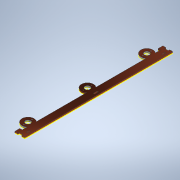
# Autodesk Inventor part: chassis_1_1
Saved by Autodesk Inventor 2022 (Build 260153000, 153)
## iProperties
Created: 2023-03-24
Part Number: chassis_1_1
Material: 一般
Document SubType Name: Modeling
Designer: Johnny Jou
Density: 1 g/cm^3
Appearance: 預設
Author: Johnny Jou
Autodesk Inventor part; units mm, degrees
ref_plane "YZ Plane" through (0, 0, 0) normal (1, 0, 0) x (0, 1, 0)
ref_plane "XZ Plane" through (0, 0, 0) normal (0, 1, 0) x (-1, 0, 0)
ref_plane "XY Plane" through (0, 0, 0) normal (0, 0, 1) x (1, 0, 0)
sketch "草圖1" plane through (0, 0, 0) normal (0, 1, 0) x (-1, 0, 0)
  line L0 (0, 0) -> (0, -306)
  arc A0 (15, -162.6047) -> (15, -143.3953) centre (23, -153) ccw
  circle A1 centre (23, -153) radius 26 construction
  line L1 (15, -296) -> (15, -162.6047)
  line L2 (15, -143.3953) -> (15, -10)
  circle A2 centre (23, -144.5) radius 1
  circle A3 centre (23, -161.5) radius 1
  line L3 (20, 0) -> (20, -10)
  line L4 (20, -10) -> (15, -10)
  line L5 (0, -10) -> (0, 0)
  line L6 (6, 0) -> (6, -3)
  line L7 (6, -3) -> (14, -3)
  line L8 (14, -3) -> (14, 0)
  line L9 (0, 0) -> (6, 0)
  line L10 (14, 0) -> (20, 0)
  line L11 (15, 0) -> (14, 0)
  line L12 (6, 0) -> (0, 0)
  line L13 (20, -306) -> (20, -296)
  line L14 (20, -296) -> (15, -296)
  line L15 (0, -290) -> (0, -306)
  line L16 (6, -306) -> (6, -303)
  line L17 (6, -303) -> (14, -303)
  line L18 (14, -303) -> (14, -306)
  line L19 (0, -306) -> (6, -306)
  line L20 (14, -306) -> (20, -306)
  dimension "d1" = 15
  dimension "d2" = 25
  dimension "d3" = 52
  dimension "d4" = 23
  dimension "d6" = 2
  dimension "d7" = 17
  dimension "d8" = 8.5
  dimension "d9" = 10
  dimension "d10" = 20
  dimension "d11" = 8
  dimension "d12" = 3
  dimension "d13" = 6
  dimension "d15" = 3
  dimension "d16" = 8
  dimension "d17" = 6
  dimension "d34" = 306
  dimension "d35" = 153
  dimension "d36" = 10
  dimension "d55" = 8.5
  constraints: 42 end point, 10 parallel, 6 horizontal, 6 perpendicular, 4 centre point, 2 coincident, 2 collinear, 2 point on circle, 1 equal radius, 1 vertical alignment
  measures "d1" distance of L11.start L0.start
  measures "d2" diameter of A0
  measures "d3" diameter of A1
  measures "d4" distance from line of L0 A0.centre
  measures "d6" diameter of A2
  measures "d7" distance of A3.centre A2.centre
  measures "d8" distance of A0.centre A3.centre
  measures "d9" distance of L3.start L3.end
  measures "d10" distance between parallel lines of L0 L3
  measures "d11" distance of L6.end L7.end
  measures "d12" distance of L7.end L8.end
  measures "d13" distance between parallel lines of L5 L6
  measures "d15" distance of L17.end L18.end
  measures "d16" distance of L16.end L17.end
  measures "d17" distance between parallel lines of L0 L16
  measures "d34" distance of L0.start L0.end
  measures "d35" distance from line of L19 A0.centre
  measures "d36" distance of L13.start L13.end
  measures "d55" distance of A0.centre A2.centre
extrude "擠出1" add sketch "草圖1" along normal blind 3
sketch "草圖2" plane through (0, 3, 0) normal (0, 1, 0) x (1, 0, 0)
  line L0 (-7, 149) -> (-4, 149)
  line L1 (-4, 149) -> (-4, 157)
  line L2 (-4, 157) -> (-7, 157)
  line L3 (-7, 157) -> (-7, 149)
  arc A0 (-15, 162.6047) -> (-15, 143.3953) centre (-23, 153) ccw projected
  line L4 (-15, 143.3953) -> (-15, 10) projected
  circle A1 centre (-23, 153) radius 12.5 construction
  line L5 (0, 0) -> (0, 306) projected
  line L6 (-7, 10) -> (-4, 10)
  line L7 (-4, 10) -> (-4, 16)
  line L8 (-4, 16) -> (-7, 16)
  line L9 (-7, 16) -> (-7, 10)
  line L10 (-14, 3) -> (-6, 3) projected
  line L11 (-7, 290) -> (-4, 290)
  line L12 (-4, 290) -> (-4, 296)
  line L13 (-4, 296) -> (-7, 296)
  line L14 (-7, 296) -> (-7, 290)
  line L15 (-6, 303) -> (-14, 303) projected
  dimension "d20" = 8
  dimension "d21" = 3
  dimension "d22" = 4
  dimension "d23" = 4
  dimension "d24" = 6
  dimension "d25" = 3
  dimension "d26" = 4
  dimension "d27" = 7
  dimension "d28" = 6
  dimension "d29" = 3
  dimension "d30" = 4
  dimension "d31" = 7
  constraints: 24 end point, 6 parallel, 3 horizontal, 3 perpendicular, 1 coincident, 3 other
  measures "d20" distance of L2.end L0.start
  measures "d21" distance of L1.end L2.end
  measures "d22" distance from line of A0.centre L2
  measures "d23" distance between parallel lines of L5 L1
  measures "d24" distance of L8.end L6.start
  measures "d25" distance of L7.end L8.end
  measures "d26" distance between parallel lines of L5 L7
  measures "d27" distance between parallel lines of L10 L6
  measures "d28" distance of L13.end L11.start
  measures "d29" distance of L11.start L11.end
  measures "d30" distance between parallel lines of L5 L12
  measures "d31" distance between parallel lines of L15 L13
extrude "擠出2" cut sketch "草圖2" against normal up to surface (3 mm away)
sketch "草圖3" plane through (0, 3, 0) normal (0, 1, 0) x (1, 0, 0)
  arc A0 (-15, 162.6047) -> (-15, 143.3953) centre (-23, 153) ccw projected
  circle A1 centre (-23, 153) radius 5.5
  point P0 (0, 0)
  dimension "d37" = 11
  constraints: 1 centre point, 1 coincident
  measures "d37" diameter of A1
extrude "擠出3" cut sketch "草圖3" against normal up to surface (3 mm away)
sketch "草圖4" plane through (0, 3, 0) normal (0, 1, 0) x (1, 0, 0)
  circle A0 centre (-23, 153) radius 5.5 projected
  arc A1 (-15, 162.6047) -> (-15, 143.3953) centre (-23, 153) ccw projected
  circle A2 centre (-23, 144.5) radius 1 projected
  circle A3 centre (-23, 161.5) radius 1 projected
  circle A4 centre (-23, 30) radius 12.5
  circle A5 centre (-23, 30) radius 5.5
  circle A6 centre (-23, 38.5) radius 1
  circle A7 centre (-23, 21.5) radius 1
  line L0 (-15, 143.3953) -> (-15, 10) projected
  circle A8 centre (-23, 276) radius 12.5
  circle A9 centre (-23, 276) radius 5.5
  circle A10 centre (-23, 284.5) radius 1
  circle A11 centre (-23, 267.5) radius 1
  point P0 (0, 0)
  point P1 (-15, 20.3953)
  point P2 (-15, 39.6047)
  dimension "d40" = 2
  dimension "d41" = 11
  dimension "d42" = 25
  dimension "d43" = 17
  dimension "d44" = 8.5
  dimension "d45" = 123
  dimension "d48" = 246
  constraints: 8 centre point, 3 vertical alignment, 2 coincident, 1 equal radius, 1 vertical, 8 other
  measures "d40" diameter of A6
  measures "d41" diameter of A5
  measures "d42" diameter of A4
  measures "d43" distance of A7.centre A6.centre
  measures "d44" distance of A4.centre A6.centre
  measures "d45" distance of A0.centre A4.centre
  measures "d48" distance of A4.centre A8.centre
extrude "擠出4" add sketch "草圖4" against normal up to surface (3 mm away) contours L0 A4 | A8 picked at (-15.8333, 30)
sketch "草圖5" plane through (0, 0, 0) normal (0, -1, 0) x (1, 0, 0)
  circle A0 centre (-23, -267.5) radius 1 projected
  circle A1 centre (-23, -284.5) radius 1 projected
  circle A2 centre (-23, -276) radius 5.5 projected
  circle A3 centre (-23, -21.5) radius 1 projected
  circle A4 centre (-23, -38.5) radius 1 projected
  circle A5 centre (-23, -30) radius 5.5 projected
  circle A6 centre (-23, -161.5) radius 1 projected
  circle A7 centre (-23, -144.5) radius 1 projected
  line L0 (-15, -296) -> (-15, -285.6047) projected
  line L1 (-20, -296) -> (-15, -296) projected
  line L2 (-20, -306) -> (-20, -296) projected
  line L3 (-14, -306) -> (-20, -306) projected
  line L4 (-14, -303) -> (-14, -306) projected
  line L5 (-6, -303) -> (-14, -303) projected
  line L6 (-6, -306) -> (-6, -303) projected
  line L7 (0, -306) -> (-6, -306) projected
  line L8 (0, 0) -> (0, -306) projected
  line L9 (-6, 0) -> (0, 0) projected
  line L10 (-6, -3) -> (-6, 0) projected
  line L11 (-14, -3) -> (-6, -3) projected
  line L12 (-14, 0) -> (-14, -3) projected
  line L13 (-20, 0) -> (-14, 0) projected
  line L14 (-20, -10) -> (-20, 0) projected
  line L15 (-15, -10) -> (-20, -10) projected
  line L16 (-15, -20.3953) -> (-15, -10) projected
  arc A8 (-15, -20.3953) -> (-15, -39.6047) centre (-23, -30) ccw projected
  line L17 (-15, -143.3953) -> (-15, -39.6047) projected
  arc A9 (-15, -143.3953) -> (-15, -162.6047) centre (-23, -153) ccw projected
  line L18 (-15, -266.3953) -> (-15, -162.6047) projected
  arc A10 (-15, -266.3953) -> (-15, -285.6047) centre (-23, -276) ccw projected
  line L19 (-7, -149) -> (-4, -149) projected
  line L20 (-4, -149) -> (-4, -157) projected
  line L21 (-4, -157) -> (-7, -157) projected
  line L22 (-7, -157) -> (-7, -149) projected
  line L23 (-4, -10) -> (-4, -16) projected
  line L24 (-4, -16) -> (-7, -16) projected
  line L25 (-7, -16) -> (-7, -10) projected
  line L26 (-7, -10) -> (-4, -10) projected
  line L27 (-4, -290) -> (-4, -296) projected
  line L28 (-4, -296) -> (-7, -296) projected
  line L29 (-7, -296) -> (-7, -290) projected
  line L30 (-7, -290) -> (-4, -290) projected
  circle A11 centre (-23, -153) radius 5.5 projected
equation "\"d8\" = 0.5 * d7"
equation "\"d44\" = 0.5 * d43"
